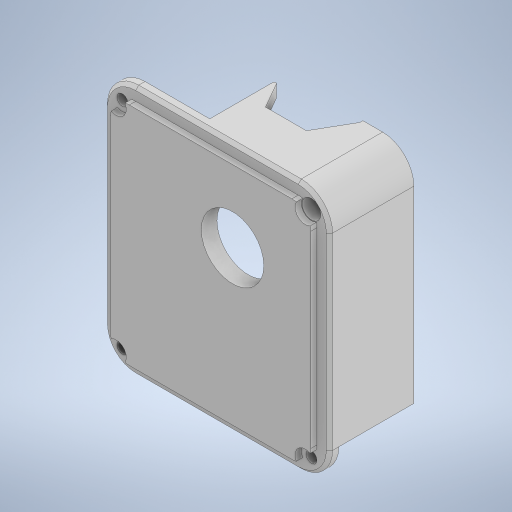
# Autodesk Inventor part: 가스벨브 하우징 커버
Saved by Autodesk Inventor 2023 (Build 270158000, 158)
## iProperties
Created: 2022-08-16
Part Number: 가스벨브 하우징 커버
Material: 일반
Document SubType Name: Modeling
Designer: fly01
Density: 1 g/cm^3
Appearance: 기본값
Author: fly01
Autodesk Inventor part; units mm, degrees
ref_plane "YZ Plane" through (0, 0, 0) normal (1, 0, 0) x (0, 1, 0)
ref_plane "XZ Plane" through (0, 0, 0) normal (0, 1, 0) x (-1, 0, 0)
ref_plane "XY Plane" through (0, 0, 0) normal (0, 0, 1) x (1, 0, 0)
sketch "스케치1" plane through (0, 0, 0) normal (0, 0, 1) x (1, 0, 0)
  line L0 (-26, 40.1) -> (26, 40.1)
  line L1 (36, 30.1) -> (36, -30.1)
  line L2 (26, -40.1) -> (-26, -40.1)
  line L3 (-36, -30.1) -> (-36, 30.1)
  line L4 (-36, 40.1) -> (36, -40.1) construction
  line L5 (36, 40.1) -> (-36, -40.1) construction
  arc A0 (-26, 40.1) -> (-36, 30.1) centre (-26, 30.1) ccw
  arc A1 (36, 30.1) -> (26, 40.1) centre (26, 30.1) ccw
  arc A2 (26, -40.1) -> (36, -30.1) centre (26, -30.1) ccw
  arc A3 (-36, -30.1) -> (-26, -40.1) centre (-26, -30.1) ccw
  line L6 (26, 36.1) -> (-26, 36.1)
  arc A4 (-26, 36.1) -> (-32, 30.1) centre (-26, 30.1) ccw
  line L7 (-32, 30.1) -> (-32, -30.1)
  arc A5 (-32, -30.1) -> (-26, -36.1) centre (-26, -30.1) ccw
  line L8 (-26, -36.1) -> (26, -36.1)
  arc A6 (26, -36.1) -> (32, -30.1) centre (26, -30.1) ccw
  line L9 (32, -30.1) -> (32, 30.1)
  arc A7 (32, 30.1) -> (26, 36.1) centre (26, 30.1) ccw
  circle A8 centre (-30.2426, 34.3426) radius 1.75
  circle A9 centre (-30.2426, 34.3426) radius 3.25
  line L10 (0, 0) -> (0, 12.3983)
  line L11 (0, 0) -> (8.6962, 0)
  circle A10 centre (30.2426, 34.3426) radius 1.75
  circle A11 centre (30.2426, 34.3426) radius 3.25
  line L12 (36, -40.1) -> (-36, 40.1) construction
  circle A12 centre (-30.2426, -34.3426) radius 1.75
  circle A13 centre (-30.2426, -34.3426) radius 3.25
  circle A14 centre (30.2426, -34.3426) radius 1.75
  circle A15 centre (30.2426, -34.3426) radius 3.25
  line L13 (-5.3, 40.1) -> (-5.3, 36.1)
  line L14 (36, -30.1) -> (32, -30.1)
  point P0 (-31.8324, 31.508)
  point P1 (-27.408, 35.9324)
  point P2 (27.408, 35.9324)
  point P3 (31.8324, 31.508)
  point P4 (31.8324, -31.508)
  point P5 (27.408, -35.9324)
  point P6 (-27.408, -35.9324)
  point P7 (-31.8324, -31.508)
  point P8 (28.838, 35.3864)
  point P9 (31.2864, 32.938)
  point P10 (32, -30.1)
  point P11 (-31.2864, -32.938)
  point P12 (-28.838, -35.3864)
  point P13 (31.2864, -32.938)
  point P14 (28.838, -35.3864)
  point P15 (-28.838, 35.3864)
  point P16 (-31.2864, 32.938)
  dimension "d0" = 72
  dimension "d1" = 80.2
  dimension "d2" = 10
  dimension "d3" = 4
  dimension "d4" = 3.5
  dimension "d5" = 6.5
  dimension "d8" = 41.3
  dimension "d11" = 10
  constraints: 30 end point, 17 point on circle, 16 centre point, 12 point on line, 8 tangent, 6 symmetric about line, 4 coincident, 4 parallel, 4 perpendicular, 3 equal radius, 2 horizontal, 2 midpoint, 1 vertical, 13 other
  measures "d0" distance of L4.start L5.start
  measures "d1" distance of L5.start L4.end
  measures "d2" radius of A0
  measures "d3" distance between parallel lines of L0 L6
  measures "d4" diameter of A8
  measures "d5" diameter of A9
  measures "d8" distance between parallel lines of L1 L13
  measures "d11" distance between parallel lines of L2 L14
extrude "돌출1" add sketch "스케치1" against normal blind 3 contours L0 L13 L6 A4 A9 L7 A5 A13 L8 A6 A15 L14 A2 L2 A3 L3 A0 | L0 A1 L1 L14 L9 A7 A11 L6 L13 | L6 A7 A11 L9 A6 A15 L8 A5 A13 L7 A4 A9 | A11 A7 A10 | A7 A10 A11 | A9 A4 A8 | A4 A8 A9 | A15 A6 A14 | A6 A14 A15 | A13 A5 A12 | A5 A12 A13
extrude "돌출2" add sketch "스케치1" along normal blind 2 contours L6 A7 A11 L9 A6 A15 L8 A5 A13 L7 A4 A9
extrude "돌출3" add sketch "스케치1" against normal blind 27 contours L0 A1 L1 L14 L9 A7 A11 L6 L13 | A11 A7 A10 | A7 A10 A11
sketch "스케치2" plane through (0, 0, 0) normal (0, 0, 1) x (1, 0, 0)
  circle A0 centre (30.2426, 34.3426) radius 1.75 projected
  circle A1 centre (30.2426, 34.3426) radius 3
  point P0 (0, 0)
  dimension "d14" = 6
  constraints: 1 centre point, 1 coincident
  measures "d14" diameter of A1
extrude "돌출4" cut sketch "스케치2" against normal blind 22
sketch "스케치3" plane through (-26, 40.1, 0) normal (0, 1, 0) x (1, 0, 0)
  line L0 (20.7, 3) -> (20.7, 27) projected
  line L1 (20.7, 26) -> (26.95, 36.8253)
  line L2 (26.95, 36.8253) -> (39.45, 36.8253)
  line L3 (39.45, 36.8253) -> (45.7, 26)
  line L4 (45.7, 26) -> (39.45, 15.1747)
  line L5 (39.45, 15.1747) -> (26.95, 15.1747)
  line L6 (26.95, 15.1747) -> (20.7, 26)
  line L7 (20.7, 27) -> (52, 27) projected
  line L8 (45.7, 26) -> (45.7, 27)
  line L9 (20.1226, 26) -> (26.6613, 37.3253)
  line L10 (26.6613, 37.3253) -> (39.7387, 37.3253)
  line L11 (39.7387, 37.3253) -> (46.2774, 26)
  line L12 (46.2774, 26) -> (39.7387, 14.6747)
  line L13 (39.7387, 14.6747) -> (26.6613, 14.6747)
  line L14 (26.6613, 14.6747) -> (20.1226, 26)
  line L15 (26.95, 15.1747) -> (26.3726, 15.1747)
  point P0 (26, 0)
  point P1 (33.2, 26)
  point P2 (20.7, 25)
  dimension "d17" = 25
  dimension "d18" = 1
  dimension "d21" = 0.5
  constraints: 28 end point, 3 point on line, 2 horizontal, 1 perpendicular, 18 other
  measures "d17" distance of L3.end L1.start
  measures "d18" distance from line of L7 point (33.2, 26)
  measures "d21" distance between parallel lines of L6 L14
extrude "돌출5" cut sketch "스케치3" against normal blind 22 contours L6 L15 L14 L0 | L0 L7 L1 | L1 L7 L3 L4 L5 L6 | L7 L8 L3
fillet "모깎기1" radius 0.5 1 edges at (-5.3, 38.1, -25)
sketch "스케치4" plane through (0, 0, -3) normal (0, 0, -1) x (-1, 0, 0)
  line L0 (-32, -30.1) -> (-36, -30.1) projected
  arc A0 (-36, -30.1) -> (-26, -40.1) centre (-26, -30.1) ccw projected
  line L1 (-26, -40.1) -> (26, -40.1) projected
  arc A1 (26, -40.1) -> (36, -30.1) centre (26, -30.1) ccw projected
  line L2 (36, -30.1) -> (36, 30.1) projected
  arc A2 (36, 30.1) -> (26, 40.1) centre (26, 30.1) ccw projected
  line L3 (26, 40.1) -> (5.3, 40.1) projected
  line L4 (5.3, 40.1) -> (5.3, 36.1) projected
  line L5 (5.3, 36.1) -> (-26, 36.1) projected
  arc A3 (-26, 36.1) -> (-27.408, 35.9324) centre (-26, 30.1) ccw projected
  arc A4 (-31.8324, 31.508) -> (-27.408, 35.9324) centre (-30.2426, 34.3426) ccw projected
  arc A5 (-31.8324, 31.508) -> (-32, 30.1) centre (-26, 30.1) ccw projected
  line L6 (-32, 30.1) -> (-32, -30.1) projected
  circle A6 centre (30.2426, 34.3426) radius 1.75 projected
  circle A7 centre (30.2426, -34.3426) radius 1.75 projected
  circle A8 centre (-30.2426, -34.3426) radius 1.75 projected
  line L7 (26, -36.1) -> (-26, -36.1)
  arc A9 (-30.4721, -34.1) -> (-26, -36.1) centre (-26, -30.1) ccw
  line L8 (-30.4721, -34.1) -> (-28, -34.1)
  line L9 (-28, -34.1) -> (-28, 27.4482)
  arc A10 (-28, 27.4482) -> (-23.3482, 32.1) centre (-30.2426, 34.3426) ccw
  line L10 (-23.3482, 32.1) -> (9.3, 32.1)
  line L11 (9.3, 32.1) -> (9.3, 36.1)
  line L12 (9.3, 36.1) -> (26, 36.1)
  arc A11 (32, 30.1) -> (26, 36.1) centre (26, 30.1) ccw
  line L13 (32, 30.1) -> (32, -30.1)
  arc A12 (26, -36.1) -> (32, -30.1) centre (26, -30.1) ccw
  line L14 (-15.5, -36.1) -> (1.5, -36.1)
  line L15 (1.5, -36.1) -> (1.5, -40.1)
  line L16 (1.5, -40.1) -> (-15.5, -40.1)
  line L17 (-15.5, -40.1) -> (-15.5, -36.1)
  line L18 (-15.5, -36.1) -> (1.5, -40.1) construction
  line L19 (1.5, -36.1) -> (-15.5, -40.1) construction
  line L20 (-36, 30.1) -> (-36, -30.1) projected
  point P0 (0, 0)
  point P1 (-7, -38.1)
  dimension "d23" = 4
  dimension "d25" = 17
  dimension "d32" = 29
  constraints: 26 end point, 8 point on circle, 4 centre point, 2 midpoint, 2 parallel, 2 point on line, 1 horizontal, 1 perpendicular, 10 other
  measures "d23" distance between parallel lines of L1 L7
  measures "d25" distance of L14.start L14.end
  measures "d32" distance from line of L20 point (-7, -38.1)
extrude "돌출6" add sketch "스케치4" along normal blind 24 contours L17 L7 L15 L1
sketch "스케치5" plane through (-26, -40.1, 0) normal (0, -1, 0) x (1, 0, 0)
  line L0 (24.5, -27) -> (41.5, -27) projected
  circle A0 centre (33, -27) radius 8.5
  point P0 (26, 0)
  dimension "d28" = 17
  constraints: 1 centre point, 1 midpoint
  measures "d28" diameter of A0
extrude "돌출7" cut sketch "스케치5" against normal blind 24 contours A0 L0 picked at (34.0047, -24.3508)
fillet "모깎기2" radius 0.2 2 edges at (15.5, -38.1, -27) (-1.5, -38.1, -27)
sketch "스케치6" plane through (0, 0, 2) normal (0, 0, 1) x (1, 0, 0)
  circle A0 centre (7, 13.05) radius 10
  line L0 (26, 40.1) -> (-26, 40.1) projected
  line L1 (36, -30.1) -> (36, 30.1) projected
  point P0 (0, 0)
  dimension "d33" = 20
  dimension "d34" = 27.05
  dimension "d35" = 29
  constraints: 1 centre point
  measures "d33" diameter of A0
  measures "d34" distance from line of L0 A0.centre
  measures "d35" distance from line of L1 A0.centre
extrude "돌출8" cut sketch "스케치6" against normal blind 24
chamfer "모따기1" distance 1 angle 45 8 edges at (0, 40.1, 0) (-33.0711, 37.1711, 0) (-36, 0, 0) (-33.0711, -37.1711, 0) (0, -40.1, 0) (33.0711, -37.1711, 0) (36, 0, 0) (33.0711, 37.1711, 0)
